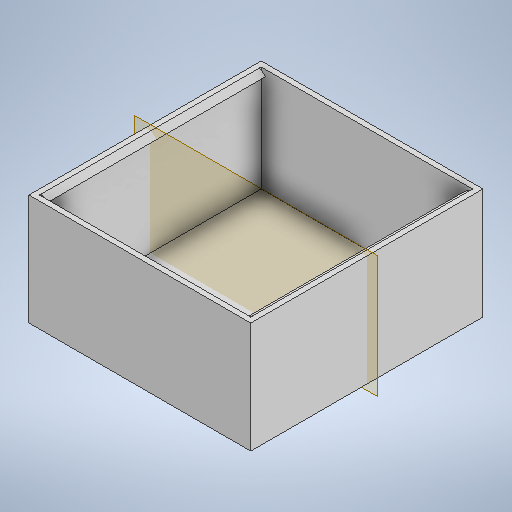
# Autodesk Inventor part: channel_base
Saved by Autodesk Inventor 2025 (Build 290162000, 162)
## iProperties
Created: 2024-08-08
Part Number: channel_base
Material: Generic
Document SubType Name: Modeling
Designer: ethan
Density: 1 g/cm^3
Appearance: Default
Author: ethan
Autodesk Inventor part; units mm, degrees
ref_plane "YZ Plane" through (0, 0, 0) normal (1, 0, 0) x (0, 1, 0)
ref_plane "XZ Plane" through (0, 0, 0) normal (0, 1, 0) x (-1, 0, 0)
ref_plane "XY Plane" through (0, 0, 0) normal (0, 0, 1) x (1, 0, 0)
sketch "Sketch1" plane through (0, 0, 0) normal (0, 0, 1) x (1, 0, 0)
  line L0 (0, 0) -> (50.8, 0)
  line L1 (50.8, 0) -> (50.8, 25.4)
  line L2 (0, 25.4) -> (0, 0)
  line L3 (1.2, 1.2) -> (49.6, 1.2)
  line L4 (49.6, 1.2) -> (49.6, 23.4)
  line L5 (1.2, 23.4) -> (1.2, 1.2)
  line L6 (50.8, 25.4) -> (49.6, 25.4)
  line L7 (1.2, 25.4) -> (0, 25.4)
  line L8 (2.614, 24.4) -> (1.2, 23.4)
  line L9 (1.2, 25.4) -> (2.614, 24.4)
  line L10 (48.186, 24.4) -> (49.6, 25.4)
  line L11 (48.186, 24.4) -> (49.6, 23.4)
  line L12 (1.2, 25.4) -> (1.2, 23.4) construction
  line L13 (1.2, 24.4) -> (2.614, 24.4) construction
  line L14 (49.6, 23.4) -> (49.6, 25.4) construction
  line L15 (49.6, 24.4) -> (48.186, 24.4) construction
  dimension "Width" = 50.8
  dimension "Height" = 25.4
  dimension "Offset" = 1.2
  dimension "LeftEdge" = 1.2
  dimension "RightEdge" = 1.2
  dimension "LT_Height" = 2
  dimension "LT_Width" = 1.414
  dimension "RT_Width" = 1.414
  dimension "RT_Height" = 2
  constraints: 32 end point, 4 parallel, 4 perpendicular, 2 midpoint, 1 horizontal, 1 vertical
  measures "Width" distance of L2.start L1.end
  measures "Height" distance of L1.end L0.end
  measures "Offset" distance between parallel lines of L2 L5
  measures "LeftEdge" distance of L7.start L2.start
  measures "RightEdge" distance of L1.end L6.end
  measures "LT_Height" distance of L7.start L5.start
  measures "LT_Width" distance of L13.start L8.start
  measures "RT_Width" distance of L15.start L10.start
  measures "RT_Height" distance of L4.end L6.end
extrude "Extrusion1" add sketch "Sketch1" along normal blind 50
sketch "Sketch2" plane through (0, 0, 50) normal (0, 0, 1) x (1, 0, 0)
  line L0 (0, 25.4) -> (0, 0) projected
  line L1 (0, 0) -> (50.8, 0) projected
  line L2 (50.8, 0) -> (50.8, 25.4) projected
  line L3 (50.8, 25.4) -> (49.6, 25.4) projected
  line L4 (49.6, 25.4) -> (48.186, 24.4) projected
  line L5 (48.186, 24.4) -> (49.6, 23.4) projected
  line L6 (49.6, 23.4) -> (49.6, 1.2) projected
  line L7 (49.6, 1.2) -> (1.2, 1.2) projected
  line L8 (1.2, 1.2) -> (1.2, 23.4) projected
  line L9 (1.2, 23.4) -> (2.614, 24.4) projected
  line L10 (2.614, 24.4) -> (1.2, 25.4) projected
  line L11 (1.2, 25.4) -> (0, 25.4) projected
  line L12 (1.2, 23.4) -> (1.2, 25.4)
  line L13 (1.2, 1.2) -> (1.2, 23.4) projected
  line L14 (49.6, 23.4) -> (49.6, 25.4)
  constraints: 4 end point, 1 collinear, 1 parallel
extrude "Extrusion2" add sketch "Sketch2" along normal blind 0.4 contours L11 L12 L8 L7 L6 L14 L3 L2 L1 L0
sketch "Sketch3" plane through (0, 0, 50.4) normal (0, 0, 1) x (1, 0, 0)
  line L0 (50.8, 0) -> (50.8, 25.4) projected
  line L1 (0, 0) -> (50.8, 0)
  line L2 (50.8, 0) -> (50.8, 25.4)
  line L3 (50.8, 25.4) -> (0, 25.4)
  line L4 (0, 25.4) -> (0, 0)
  constraints: 8 end point, 2 parallel, 1 horizontal, 1 perpendicular
ref_plane "Work Plane1" through (0, 0, 25) normal (0, 0, 1) x (1, 0, 0)
extrude "Extrusion3" add sketch "Sketch3" along normal blind 1.2
mirror "Mirror1" about plane through (0, 0, 25) normal (0, 0, 1) of "Extrusion3", "Extrusion2"
equation "\"LeftEdge\" = Offset"
equation "\"RightEdge\" = Offset"
equation "\"RT_Width\" = LT_Width"
equation "\"RT_Height\" = LT_Height"
body "Solid1"
